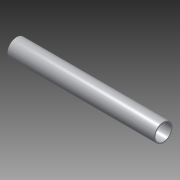
# Autodesk Inventor part: Caster Wheel Leg
Saved by Autodesk Inventor 2014 (Build 180170000, 170)
## iProperties
Created: 2014-02-25
Part Number: Caster Wheel Leg
Material: Aluminum 6061
Document SubType Name: Modeling
Designer: Nitesh
Density: 2.71 g/cm^3
Appearance: Aluminum - Flat
Mass: 8.1747 g
Surface Area: 76.5999 cm^2
Volume: 3.01649 cm^3
Author: Nitesh
Autodesk Inventor part; units mm, degrees
ref_plane "YZ Plane" through (0, 0, 0) normal (1, 0, 0) x (0, 1, 0)
ref_plane "XZ Plane" through (0, 0, 0) normal (0, 1, 0) x (-1, 0, 0)
ref_plane "XY Plane" through (0, 0, 0) normal (0, 0, 1) x (1, 0, 0)
sketch "Sketch1" plane through (0, 0, 0) normal (1, 0, 0) x (0, 1, 0)
  circle A0 centre (0, 0) radius 6.35
  circle A1 centre (0, 0) radius 5.5563
  dimension "d0" = 12.7
  dimension "d1" = 11.1125
  constraints: 2 centre point, 1 coincident
  measures "d0" diameter of A0
  measures "d1" diameter of A1
extrude "Extrusion1" add sketch "Sketch1" along normal blind 101.6
body "Solid1"
